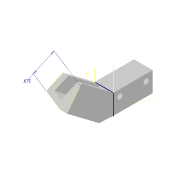
# Autodesk Inventor part: Delivery bin arm connector v2
Saved by Autodesk Inventor 2018 (Build 220112000, 112)
## iProperties
Created: 2019-01-05
Part Number: Delivery bin arm connector v2
Material: Generic
Document SubType Name: Modeling
Designer: ball
Density: 1 g/cm^3
Appearance: Default
Author: ball
Autodesk Inventor part; units mm, degrees
ref_plane "YZ Plane" through (0, 0, 0) normal (1, 0, 0) x (0, 1, 0)
ref_plane "XZ Plane" through (0, 0, 0) normal (0, 1, 0) x (-1, 0, 0)
ref_plane "XY Plane" through (0, 0, 0) normal (0, 0, 1) x (1, 0, 0)
sketch "Sketch1" plane through (0, 0, 0) normal (1, 0, 0) x (0, 1, 0)
  line L0 (0, 0) -> (14.859, 0)
  line L1 (14.859, 0) -> (14.859, 29.337)
  line L2 (14.859, 29.337) -> (0, 29.337)
  line L3 (0, 29.337) -> (0, 0)
  circle A0 centre (10.1092, 24.4475) radius 1.9685
  circle A1 centre (10.1092, 4.8895) radius 1.9685
  dimension "d0" = 14.859
  dimension "d1" = 29.337
  dimension "d2" = 3.937
  dimension "d3" = 4.8895
  dimension "d4" = 10.1092
  dimension "d5" = 3.937
  dimension "d6" = 19.558
  constraints: 8 end point, 2 centre point, 2 parallel, 1 horizontal, 1 perpendicular
  measures "d0" distance of L2.end L1.end
  measures "d1" distance of L1.end L0.end
  measures "d2" diameter of A0
  measures "d3" distance from line of A0.centre L2
  measures "d4" distance from line of L3 A0.centre
  measures "d5" diameter of A1
  measures "d6" distance of A1.centre A0.centre
extrude "Extrusion1" add sketch "Sketch1" against normal blind 13.97
ref_plane "Work Plane1" through (0, 14.859, 0) normal (0.9396926, -0.3420201, 0) x (0, 0, 1)
ref_plane "Work Plane2" through (0, 14.859, 29.337) normal (0, 0.601815, 0.7986355) x (-1, 0, 0)
sketch "Sketch5" plane through (0, 14.859, 29.337) normal (0, 0.601815, 0.7986355) x (-1, 0, 0)
  line L0 (0, 0) -> (13.97, 0) construction
  line L1 (0, 0) -> (13.97, 0)
  line L2 (13.97, 0) -> (18.6611, 12.8888)
  line L3 (13.97, 0) -> (27.686, 0) construction
  line L4 (18.6611, 12.8888) -> (5.1756, 17.7972)
  line L5 (5.1756, 17.7972) -> (0, 3.5773)
  line L6 (0, 11.8669) -> (0, -5.7885) projected
  line L7 (13.97, 0) -> (0, 0)
  line L8 (0, 0) -> (0, 3.5773)
  dimension "d35" = 13.716
  dimension "d36" = 70
  dimension "d37" = 14.351
  constraints: 14 end point, 2 collinear, 1 equal length, 1 horizontal, 1 point on line, 1 vertical
  measures "d35" distance of L0.end L2.end
  measures "d36" angle of L3 L2
  measures "d37" distance of L2.end L4.end
extrude "Extrusion4" add sketch "Sketch5" along normal blind 29.718
sketch "Sketch6" plane through (0, 32.7437, 53.0709) normal (0, 0.601815, 0.7986355) x (1, 0, 0)
  line L0 (-13.97, 0) -> (-18.6611, -12.8888) construction
  line L1 (0, 0) -> (0, -11.8669) construction
  line L2 (-13.97, -11.8669) -> (-13.97, 0) construction
  line L3 (-5.1756, -17.7972) -> (0, -3.5773) construction
  line L4 (0.6883, -1.6861) -> (-12.7972, 3.2222) construction
  line L5 (-18.6611, -12.8888) -> (-5.1756, -17.7972) construction
  point P0 (0, 5.7885)
  dimension "d40" = 17.145
  constraints: 2 end point, 2 point on line, 1 perpendicular
  measures "d40" distance between parallel lines of L5 L4
sketch "Sketch7" plane through (0, 32.7437, 53.0709) normal (0, 0.601815, 0.7986355) x (1, 0, 0)
  line L0 (0, 0) -> (-13.97, 0) projected
  line L1 (-13.97, 0) -> (-0.4845, -4.9083) construction
  line L2 (-5.1756, -17.7972) -> (0, -3.5773) projected
  line L3 (-9.9155, 0) -> (-13.7778, -10.6117)
  line L4 (-13.97, 0) -> (-18.6611, -12.8888) projected
  line L5 (-2.7525, 0) -> (-7.4528, -12.9138)
  line L6 (-13.7778, -10.6117) -> (-7.4528, -12.9138)
  line L7 (-13.97, 0) -> (-18.6611, -12.8888) projected
  line L8 (0, -3.5773) -> (0, 0) projected
  line L9 (-9.9155, 0) -> (-2.7525, 0)
  point P0 (0, 5.7885)
  point P1 (-10.3898, -1.3031)
  point P2 (-4.0647, -3.6052)
  dimension "d42" = 3.81
  dimension "d44" = 6.731
  dimension "d47" = 9.906
  constraints: 10 end point, 5 point on line, 1 horizontal, 1 parallel, 1 perpendicular
  measures "d42" distance between parallel lines of L4 L3
  measures "d44" distance between parallel lines of L5 L3
  measures "d47" distance from line of L6 L0.end
extrude "Extrusion5" cut sketch "Sketch7" against normal blind 29.718
sketch "Sketch8" plane through (-5.1756, 0.6456, 40.0476) normal (0.9396926, -0.2731494, 0.2058329) x (0, -0.601815, -0.7986355)
  line L0 (8.9424, 7.3428) -> (32.3719, 23.9335) construction
  line L1 (8.9424, 7.3428) -> (0, 1.0106) construction
  constraints: 2 end point, 1 collinear
sketch "Sketch9" plane through (-13.97, 0, 29.337) normal (0, 0, 1) x (1, 0, 0)
  line L0 (13.97, 0) -> (0, 0) projected
  line L1 (0.1922, 24.2689) -> (0.1922, 6.3841) projected
  line L2 (13.97, 0) -> (0.1922, 0)
  line L3 (0.1922, 0) -> (0.1922, 14.859)
  line L4 (13.97, 14.859) -> (13.97, 0)
  line L5 (13.97, 14.859) -> (13.97, 32.7437) projected
  line L6 (13.97, 14.859) -> (0.1922, 14.859)
  constraints: 8 end point, 2 perpendicular, 1 horizontal, 1 parallel, 1 point on line
sketch "Sketch10" plane through (0, 0, 0) normal (1, 0, 0) x (0, 0, -1)
  line L0 (0, 0) -> (-29.337, 0) projected
  line L1 (-29.337, 14.859) -> (-29.337, 0)
  line L2 (-40.0476, 0.6456) -> (-31.4898, 12.0021) projected
  line L3 (-29.337, 0) -> (-40.0476, 0.6456)
  line L4 (-31.4898, 12.0021) -> (-29.337, 14.859) projected
  line L5 (-40.0476, 0.6456) -> (-29.337, 14.859)
  constraints: 6 end point, 1 collinear, 1 vertical
extrude "Extrusion6" add sketch "Sketch10" against normal blind 13.97
sketch "Sketch11" plane through (-5.1756, 0.6456, 40.0476) normal (0, 0.601815, 0.7986355) x (1, 0, 0)
  line L0 (5.1756, 14.2199) -> (5.1756, 0) projected
  line L1 (-8.7944, 3.2009) -> (0, 0) projected
  line L2 (5.1756, 14.2199) -> (0, 0)
  line L3 (5.1756, 0) -> (0, 0) projected
  line L4 (0, 0) -> (5.1756, 0)
  line L5 (0, 0) -> (5.1756, 14.2199) projected
  line L6 (5.1756, 0) -> (5.1756, 14.2199)
  point P0 (5.1756, 23.5857)
  constraints: 6 end point, 2 collinear, 1 perpendicular
extrude "Extrusion7" add sketch "Sketch11" along normal blind 29.718
fillet "Fillet6" radius 3.175 1 edges at (-9.5728, 1.9237, 39.0844)
body "Solid1"
